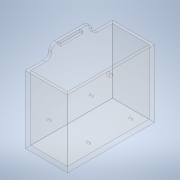
# Autodesk Inventor part: Part3
Saved by Autodesk Inventor 2022 (Build 260153000, 153)
## iProperties
Created: 2022-12-07
Part Number: Part3
Material: Polycarbonate, Clear
Document SubType Name: Modeling
Designer: S135320
Mass: 764.764 g
Surface Area: 2044.35 cm^2
Volume: 637.303 cm^3
Density: 1.2 g/cm^3
Appearance: Polycarbonate - Clear
Author: S135320
Autodesk Inventor part; units mm, degrees
ref_plane "YZ Plane" through (0, 0, 0) normal (1, 0, 0) x (0, 1, 0)
ref_plane "XZ Plane" through (0, 0, 0) normal (0, 1, 0) x (-1, 0, 0)
ref_plane "XY Plane" through (0, 0, 0) normal (0, 0, 1) x (1, 0, 0)
sketch "Sketch1" plane through (0, 0, 0) normal (0, 1, 0) x (-1, 0, 0)
  line L0 (0, 0) -> (82.55, 0)
  line L1 (82.55, 0) -> (82.55, -184.15)
  line L2 (82.55, -184.15) -> (0, -184.15)
  line L3 (0, -184.15) -> (0, 0)
  line L4 (88.9, -190.5) -> (88.9, 6.35)
  line L5 (88.9, 6.35) -> (-6.35, 6.35)
  line L6 (-6.35, 6.35) -> (-6.35, -190.5)
  line L7 (-6.35, -190.5) -> (88.9, -190.5)
  dimension "d0" = 184.15
  dimension "d1" = 82.55
  dimension "d2" = 6.35
  constraints: 16 end point, 4 parallel, 2 perpendicular, 1 horizontal, 3 other
  measures "d0" distance of L0.end L1.end
  measures "d1" distance of L0.start L0.end
  measures "d2" distance between parallel lines of L4 L1
extrude "Extrusion1" add sketch "Sketch1" along normal blind 6.35 contours L0 L1 L2 L3
extrude "Extrusion2" add sketch "Sketch1" along normal blind 152.4
sketch "Sketch2" plane through (-88.9, 0, -190.5) normal (-1, 0, 0) x (0, 0, 1)
  line L0 (53.0182, 127) -> (143.8318, 127)
  line L1 (143.8318, 127) -> (143.8318, 177.8)
  line L2 (143.8318, 177.8) -> (53.0182, 177.8)
  line L3 (53.0182, 177.8) -> (53.0182, 127)
  line L4 (190.5, 152.4) -> (6.35, 152.4) projected
  line L5 (53.0182, 127) -> (143.8318, 177.8) construction
  line L6 (143.8318, 127) -> (53.0182, 177.8) construction
  point P0 (190.5, 0)
  point P1 (98.425, 152.4)
  point P2 (53.0182, 152.4)
  point P3 (143.8318, 152.4)
  dimension "d14" = 25.4
  constraints: 12 end point, 3 midpoint, 2 parallel, 1 horizontal, 1 perpendicular
  measures "d14" distance between parallel lines of L2 L4
extrude "Extrusion3" add sketch "Sketch2" against normal blind 6.35 contours L3 L2 L1 L4
fillet "Fillet1" radius 12.7 4 edges at (-85.725, 177.8, -46.6682) (-85.725, 152.4, -46.6682) (-85.725, 177.8, -137.4818) (-85.725, 152.4, -137.4818)
sketch "Sketch3" plane through (-82.55, 6.35, 0) normal (1, 0, 0) x (0, 0, -1)
  line L0 (124.7818, 171.45) -> (59.3682, 171.45) projected
  line L1 (92.075, 171.45) -> (92.075, 193.6256)
  line L2 (67.0657, 165.1) -> (117.0843, 165.1)
  line L3 (117.0843, 165.1) -> (117.0843, 160.109)
  line L4 (117.0843, 160.109) -> (67.0657, 160.109)
  line L5 (67.0657, 160.109) -> (67.0657, 165.1)
  line L6 (67.0657, 165.1) -> (117.0843, 160.109) construction
  line L7 (117.0843, 165.1) -> (67.0657, 160.109) construction
  point P0 (0, -6.35)
  point P1 (92.075, 162.6045)
  dimension "d15" = 6.35
  constraints: 14 end point, 3 midpoint, 2 parallel, 1 horizontal, 1 perpendicular, 1 point on line, 1 vertical
  measures "d15" distance between parallel lines of L0 L2
extrude "Extrusion4" cut sketch "Sketch3" against normal blind 6.35
sketch "Sketch4" plane through (6.35, 0, 6.35) normal (1, 0, 0) x (0, 0, -1)
  line L0 (0, 152.4) -> (196.85, 152.4) projected
  line L1 (98.425, 152.4) -> (98.425, 129.719)
  circle A0 centre (98.425, 141.0595) radius 4.0936
  point P0 (6.35, 0)
  constraints: 2 end point, 2 midpoint, 1 centre point, 1 vertical
extrude "Extrusion5" cut sketch "Sketch4" against normal up to surface (6.35 mm away)
sketch "Sketch5" plane through (6.35, 0, 6.35) normal (1, 0, 0) x (0, 0, -1)
  line L0 (196.85, 0) -> (196.85, 152.4) projected
  line L1 (0, 0) -> (196.85, 0)
  line L2 (196.85, 0) -> (196.85, 31.75)
  line L3 (196.85, 31.75) -> (0, 31.75)
  line L4 (0, 31.75) -> (0, 0)
  line L5 (0, 31.75) -> (62.6052, 31.75)
  line L6 (0, 31.75) -> (50.8, 31.75)
  line L7 (196.85, 31.75) -> (146.05, 31.75)
  circle A0 centre (50.8, 31.75) radius 2.0701
  circle A1 centre (146.05, 31.75) radius 2.0701
  point P0 (6.35, 0)
  dimension "d16" = 31.75
  dimension "d17" = 50.8
  dimension "d18" = 50.8
  dimension "d19" = 4.1402
  dimension "d20" = 4.1402
  constraints: 14 end point, 4 point on line, 2 centre point, 2 coincident, 2 parallel, 1 horizontal, 1 perpendicular
  measures "d16" distance between parallel lines of L1 L3
  measures "d17" distance of L3.end L6.end
  measures "d18" distance of L2.end L7.end
  measures "d19" diameter of A1
  measures "d20" diameter of A0
extrude "Extrusion6" cut sketch "Sketch5" against normal through all contours A1 L3 | L3 A1 | A0 L3 | L3 A0
body "Solid1"
